Autodesk Inventor part; units mm, degrees
(part 2 of 2)
  line L934 (17.3523, 0.525) -> (17.2918, 0.4645)
  line L935 (17.2918, 0.4645) -> (17.2697, 0.3818)
  line L936 (17.2697, 0.3818) -> (17.2918, 0.2991)
  line L937 (17.2918, 0.2991) -> (17.3523, 0.2386)
  line L938 (17.3523, 0.2386) -> (17.435, 0.2164)
  line L939 (17.435, 0.2164) -> (17.5177, 0.2386)
  line L940 (17.5177, 0.2386) -> (17.5782, 0.2991)
  line L941 (17.5782, 0.2991) -> (17.6003, 0.3818)
  line L942 (14.4188, -4.4542) -> (14.3966, -4.3715)
  line L943 (14.3966, -4.3715) -> (14.3361, -4.311)
  line L944 (14.3361, -4.311) -> (14.2534, -4.2889)
  line L945 (14.2534, -4.2889) -> (14.1708, -4.311)
  line L946 (14.1708, -4.311) -> (14.1102, -4.3715)
  line L947 (14.1102, -4.3715) -> (14.0881, -4.4542)
  line L948 (14.0881, -4.4542) -> (14.1102, -4.5369)
  line L949 (14.1102, -4.5369) -> (14.1708, -4.5974)
  line L950 (14.1708, -4.5974) -> (14.2534, -4.6195)
  line L951 (14.2534, -4.6195) -> (14.3361, -4.5974)
  line L952 (14.3361, -4.5974) -> (14.3966, -4.5369)
  line L953 (14.3966, -4.5369) -> (14.4188, -4.4542)
  line L954 (17.4731, -10.5628) -> (17.4509, -10.4801)
  line L955 (17.4509, -10.4801) -> (17.3904, -10.4196)
  line L956 (17.3904, -10.4196) -> (17.3077, -10.3975)
  line L957 (17.3077, -10.3975) -> (17.2251, -10.4196)
  line L958 (17.2251, -10.4196) -> (17.1645, -10.4801)
  line L959 (17.1645, -10.4801) -> (17.1424, -10.5628)
  line L960 (17.1424, -10.5628) -> (17.1645, -10.6455)
  line L961 (17.1645, -10.6455) -> (17.2251, -10.706)
  line L962 (17.2251, -10.706) -> (17.3077, -10.7282)
  line L963 (17.3077, -10.7282) -> (17.3904, -10.706)
  line L964 (17.3904, -10.706) -> (17.4509, -10.6455)
  line L965 (17.4509, -10.6455) -> (17.4731, -10.5628)
  line L966 (14.546, -12.599) -> (14.5239, -12.5163)
  line L967 (14.5239, -12.5163) -> (14.4634, -12.4558)
  line L968 (14.4634, -12.4558) -> (14.3807, -12.4337)
  line L969 (14.3807, -12.4337) -> (14.298, -12.4558)
  line L970 (14.298, -12.4558) -> (14.2375, -12.5163)
  line L971 (14.2375, -12.5163) -> (14.2154, -12.599)
  line L972 (14.2154, -12.599) -> (14.2375, -12.6817)
  line L973 (14.2375, -12.6817) -> (14.298, -12.7422)
  line L974 (14.298, -12.7422) -> (14.3807, -12.7644)
  line L975 (14.3807, -12.7644) -> (14.4634, -12.7422)
  line L976 (14.4634, -12.7422) -> (14.5239, -12.6817)
  line L977 (14.5239, -12.6817) -> (14.546, -12.599)
  line L978 (15.5706, -6.8563) -> (15.5101, -6.9168)
  line L979 (15.5101, -6.9168) -> (15.488, -6.9995)
  line L980 (15.488, -6.9995) -> (15.5101, -7.0821)
  line L981 (15.5101, -7.0821) -> (15.5706, -7.1426)
  line L982 (15.5706, -7.1426) -> (15.6533, -7.1648)
  line L983 (15.6533, -7.1648) -> (15.736, -7.1426)
  line L984 (15.736, -7.1426) -> (15.7965, -7.0821)
  line L985 (15.7965, -7.0821) -> (15.8187, -6.9995)
  line L986 (17.0913, -12.09) -> (17.0691, -12.0073)
  line L987 (17.0691, -12.0073) -> (17.0086, -11.9468)
  line L988 (17.0086, -11.9468) -> (16.9259, -11.9246)
  line L989 (16.9259, -11.9246) -> (16.8433, -11.9468)
  line L990 (16.8433, -11.9468) -> (16.7828, -12.0073)
  line L991 (16.7828, -12.0073) -> (16.7606, -12.09)
  line L992 (16.7606, -12.09) -> (16.7828, -12.1726)
  line L993 (16.7828, -12.1726) -> (16.8433, -12.2332)
  line L994 (16.8433, -12.2332) -> (16.9259, -12.2553)
  line L995 (16.9259, -12.2553) -> (17.0086, -12.2332)
  line L996 (17.0086, -12.2332) -> (17.0691, -12.1726)
  line L997 (17.0691, -12.1726) -> (17.0913, -12.09)
  line L998 (17.3458, -13.6171) -> (17.3237, -13.5344)
  line L999 (17.3237, -13.5344) -> (17.2631, -13.4739)
  line L1000 (17.2631, -13.4739) -> (17.1805, -13.4518)
  line L1001 (17.1805, -13.4518) -> (17.0978, -13.4739)
  line L1002 (17.0978, -13.4739) -> (17.0373, -13.5344)
  line L1003 (17.0373, -13.5344) -> (17.0151, -13.6171)
  line L1004 (17.0151, -13.6171) -> (17.0373, -13.6998)
  line L1005 (17.0373, -13.6998) -> (17.0978, -13.7603)
  line L1006 (17.0978, -13.7603) -> (17.1805, -13.7825)
  line L1007 (17.1805, -13.7825) -> (17.2631, -13.7603)
  line L1008 (17.2631, -13.7603) -> (17.3237, -13.6998)
  line L1009 (17.3237, -13.6998) -> (17.3458, -13.6171)
  line L1010 (11.2372, -15.3988) -> (11.215, -15.3161)
  line L1011 (11.215, -15.3161) -> (11.1545, -15.2556)
  line L1012 (11.1545, -15.2556) -> (11.0719, -15.2335)
  line L1013 (11.0719, -15.2335) -> (10.9892, -15.2556)
  line L1014 (10.9892, -15.2556) -> (10.9287, -15.3161)
  line L1015 (10.9287, -15.3161) -> (10.9065, -15.3988)
  line L1016 (10.9065, -15.3988) -> (10.9287, -15.4815)
  line L1017 (10.9287, -15.4815) -> (10.9892, -15.542)
  line L1018 (10.9892, -15.542) -> (11.0719, -15.5641)
  line L1019 (11.0719, -15.5641) -> (11.1545, -15.542)
  line L1020 (11.1545, -15.542) -> (11.215, -15.4815)
  line L1021 (11.215, -15.4815) -> (11.2372, -15.3988)
  line L1022 (6.6557, -17.435) -> (6.6336, -17.3523)
  line L1023 (6.6336, -17.3523) -> (6.5731, -17.2918)
  line L1024 (6.5731, -17.2918) -> (6.4904, -17.2697)
  line L1025 (6.4904, -17.2697) -> (6.4077, -17.2918)
  line L1026 (6.4077, -17.2918) -> (6.3472, -17.3523)
  line L1027 (6.3472, -17.3523) -> (6.3251, -17.435)
  line L1028 (6.3251, -17.435) -> (6.3472, -17.5177)
  line L1029 (6.3472, -17.5177) -> (6.4077, -17.5782)
  line L1030 (6.4077, -17.5782) -> (6.4904, -17.6003)
  line L1031 (6.4904, -17.6003) -> (6.5731, -17.5782)
  line L1032 (6.5731, -17.5782) -> (6.6336, -17.5177)
  line L1033 (6.6336, -17.5177) -> (6.6557, -17.435)
  line L1034 (4.1105, -17.435) -> (4.0883, -17.3523)
  line L1035 (4.0883, -17.3523) -> (4.0278, -17.2918)
  line L1036 (4.0278, -17.2918) -> (3.9451, -17.2697)
  line L1037 (3.9451, -17.2697) -> (3.8625, -17.2918)
  line L1038 (3.8625, -17.2918) -> (3.802, -17.3523)
  line L1039 (3.802, -17.3523) -> (3.7798, -17.435)
  line L1040 (3.7798, -17.435) -> (3.802, -17.5177)
  line L1041 (3.802, -17.5177) -> (3.8625, -17.5782)
  line L1042 (3.8625, -17.5782) -> (3.9451, -17.6003)
  line L1043 (3.9451, -17.6003) -> (4.0278, -17.5782)
  line L1044 (4.0278, -17.5782) -> (4.0883, -17.5177)
  line L1045 (4.0883, -17.5177) -> (4.1105, -17.435)
  line L1046 (1.7976, -17.3523) -> (1.7371, -17.2918)
  line L1047 (1.7371, -17.2918) -> (1.6544, -17.2697)
  line L1048 (1.6544, -17.2697) -> (1.5717, -17.2918)
  line L1049 (1.5717, -17.2918) -> (1.5112, -17.3523)
  line L1050 (1.5112, -17.3523) -> (1.4891, -17.435)
  line L1051 (1.4891, -17.435) -> (1.5112, -17.5177)
  line L1052 (1.5112, -17.5177) -> (1.5717, -17.5782)
  line L1053 (1.5717, -17.5782) -> (1.6544, -17.6003)
  line L1054 (1.6544, -17.6003) -> (1.7371, -17.5782)
  line L1055 (1.7371, -17.5782) -> (1.7976, -17.5177)
  line L1056 (1.7976, -17.5177) -> (1.8198, -17.435)
  line L1057 (-4.117, -17.5782) -> (-4.0565, -17.5177)
  line L1058 (-4.0565, -17.5177) -> (-4.0343, -17.435)
  line L1059 (-1.7436, -17.435) -> (-1.7658, -17.3523)
  line L1060 (-1.7658, -17.3523) -> (-1.8263, -17.2918)
  line L1061 (-1.8263, -17.2918) -> (-1.9089, -17.2697)
  line L1062 (-1.9089, -17.2697) -> (-1.9916, -17.2918)
  line L1063 (-1.9916, -17.2918) -> (-2.0521, -17.3523)
  line L1064 (-2.0521, -17.3523) -> (-2.0743, -17.435)
  line L1065 (-2.0743, -17.435) -> (-2.0521, -17.5177)
  line L1066 (-2.0521, -17.5177) -> (-1.9916, -17.5782)
  line L1067 (-1.9916, -17.5782) -> (-1.9089, -17.6003)
  line L1068 (-1.9089, -17.6003) -> (-1.8263, -17.5782)
  line L1069 (-1.8263, -17.5782) -> (-1.7658, -17.5177)
  line L1070 (-1.7658, -17.5177) -> (-1.7436, -17.435)
  line L1071 (-5.816, -15.6533) -> (-5.8382, -15.5706)
  line L1072 (-5.8382, -15.5706) -> (-5.8987, -15.5101)
  line L1073 (-5.8987, -15.5101) -> (-5.9813, -15.488)
  line L1074 (-5.9813, -15.488) -> (-6.064, -15.5101)
  line L1075 (-6.064, -15.5101) -> (-6.1245, -15.5706)
  line L1076 (-6.1245, -15.5706) -> (-6.1467, -15.6533)
  line L1077 (-6.1467, -15.6533) -> (-6.1245, -15.736)
  line L1078 (-6.1245, -15.736) -> (-6.064, -15.7965)
  line L1079 (-6.064, -15.7965) -> (-5.9813, -15.8187)
  line L1080 (-5.9813, -15.8187) -> (-5.8987, -15.7965)
  line L1081 (-5.8987, -15.7965) -> (-5.8382, -15.736)
  line L1082 (-5.8382, -15.736) -> (-5.816, -15.6533)
  line L1083 (-8.8703, -14.8897) -> (-8.8925, -14.8071)
  line L1084 (-8.8925, -14.8071) -> (-8.953, -14.7466)
  line L1085 (-8.953, -14.7466) -> (-9.0357, -14.7244)
  line L1086 (-9.0357, -14.7244) -> (-9.1183, -14.7466)
  line L1087 (-9.1183, -14.7466) -> (-9.1788, -14.8071)
  line L1088 (-9.201, -14.8897) -> (-9.1788, -14.9724)
  line L1089 (-9.1788, -14.9724) -> (-9.1183, -15.0329)
  line L1090 (-9.1183, -15.0329) -> (-9.0357, -15.0551)
  line L1091 (-9.0357, -15.0551) -> (-8.953, -15.0329)
  line L1092 (-8.953, -15.0329) -> (-8.8925, -14.9724)
  line L1093 (-8.8925, -14.9724) -> (-8.8703, -14.8897)
  line L1094 (-11.6701, -14.8897) -> (-11.6922, -14.8071)
  line L1095 (-11.6922, -14.8071) -> (-11.7528, -14.7466)
  line L1096 (-11.7528, -14.7466) -> (-11.8354, -14.7244)
  line L1097 (-11.8354, -14.7244) -> (-11.9181, -14.7466)
  line L1098 (-11.9181, -14.7466) -> (-11.9786, -14.8071)
  line L1099 (-11.9786, -14.8071) -> (-12.0008, -14.8897)
  line L1100 (-12.0008, -14.8897) -> (-11.9786, -14.9724)
  line L1101 (-11.9786, -14.9724) -> (-11.9181, -15.0329)
  line L1102 (-11.9181, -15.0329) -> (-11.8354, -15.0551)
  line L1103 (-11.8354, -15.0551) -> (-11.7528, -15.0329)
  line L1104 (-11.7528, -15.0329) -> (-11.6922, -14.9724)
  line L1105 (-11.6922, -14.9724) -> (-11.6701, -14.8897)
  line L1106 (-13.4739, -15.8252) -> (-13.5344, -15.7647)
  line L1107 (-13.6998, -15.7647) -> (-13.7603, -15.8252)
  line L1108 (-13.7603, -15.8252) -> (-13.7825, -15.9078)
  line L1109 (-13.7825, -15.9078) -> (-13.7603, -15.9905)
  line L1110 (-13.7603, -15.9905) -> (-13.6998, -16.051)
  line L1111 (-13.6998, -16.051) -> (-13.6171, -16.0732)
  line L1112 (-13.6171, -16.0732) -> (-13.5344, -16.051)
  line L1113 (-13.5344, -16.051) -> (-13.4739, -15.9905)
  line L1114 (-13.4739, -15.9905) -> (-13.4518, -15.9078)
  line L1115 (-14.9789, -17.3077) -> (-15.0011, -17.2251)
  line L1116 (-15.0011, -17.2251) -> (-15.0616, -17.1645)
  line L1117 (-15.0616, -17.1645) -> (-15.1443, -17.1424)
  line L1118 (-15.1443, -17.1424) -> (-15.2269, -17.1645)
  line L1119 (-15.2269, -17.1645) -> (-15.2875, -17.2251)
  line L1120 (-15.2875, -17.2251) -> (-15.3096, -17.3077)
  line L1121 (-15.3096, -17.3077) -> (-15.2875, -17.3904)
  line L1122 (-15.2875, -17.3904) -> (-15.2269, -17.4509)
  line L1123 (-15.2269, -17.4509) -> (-15.1443, -17.4731)
  line L1124 (-15.1443, -17.4731) -> (-15.0616, -17.4509)
  line L1125 (-15.0616, -17.4509) -> (-15.0011, -17.3904)
  line L1126 (-15.0011, -17.3904) -> (-14.9789, -17.3077)
  line L1127 (-17.5177, -14.6193) -> (-17.5782, -14.6798)
  line L1128 (-17.5782, -14.6798) -> (-17.6003, -14.7625)
  line L1129 (-17.5782, -14.8452) -> (-17.5177, -14.9057)
  line L1130 (-17.5177, -14.9057) -> (-17.435, -14.9278)
  line L1131 (-17.435, -14.9278) -> (-17.3523, -14.9057)
  line L1132 (-17.3523, -14.9057) -> (-17.2918, -14.8452)
  line L1133 (-17.2918, -14.8452) -> (-17.2697, -14.7625)
  line L1134 (-15.488, -13.3626) -> (-15.5101, -13.2799)
  line L1135 (-15.5101, -13.2799) -> (-15.5706, -13.2194)
  line L1136 (-15.5706, -13.2194) -> (-15.6533, -13.1972)
  line L1137 (-15.6533, -13.1972) -> (-15.736, -13.2194)
  line L1138 (-15.736, -13.2194) -> (-15.7965, -13.2799)
  line L1139 (-15.7965, -13.2799) -> (-15.8187, -13.3626)
  line L1140 (-15.8187, -13.3626) -> (-15.7965, -13.4453)
  line L1141 (-15.6533, -13.5279) -> (-15.5706, -13.5058)
  line L1142 (-15.5706, -13.5058) -> (-15.5101, -13.4453)
  line L1143 (-15.5101, -13.4453) -> (-15.488, -13.3626)
  line L1144 (-14.9789, -11.5809) -> (-15.0011, -11.4982)
  line L1145 (-15.0011, -11.4982) -> (-15.0616, -11.4377)
  line L1146 (-15.0616, -11.4377) -> (-15.1443, -11.4156)
  line L1147 (-15.1443, -11.4156) -> (-15.2269, -11.4377)
  line L1148 (-15.2269, -11.4377) -> (-15.2875, -11.4982)
  line L1149 (-15.2875, -11.4982) -> (-15.3096, -11.5809)
  line L1150 (-15.3096, -11.5809) -> (-15.2875, -11.6636)
  line L1151 (-15.2875, -11.6636) -> (-15.2269, -11.7241)
  line L1152 (-15.2269, -11.7241) -> (-15.1443, -11.7463)
  line L1153 (-15.1443, -11.7463) -> (-15.0616, -11.7241)
  line L1154 (-15.0616, -11.7241) -> (-15.0011, -11.6636)
  line L1155 (-15.0011, -11.6636) -> (-14.9789, -11.5809)
  line L1156 (-14.7244, -8.7811) -> (-14.7466, -8.6985)
  line L1157 (-14.7466, -8.6985) -> (-14.8071, -8.6379)
  line L1158 (-14.8071, -8.6379) -> (-14.8897, -8.6158)
  line L1159 (-14.8897, -8.6158) -> (-14.9724, -8.6379)
  line L1160 (-14.9724, -8.6379) -> (-15.0329, -8.6985)
  line L1161 (-15.0329, -8.6985) -> (-15.0551, -8.7811)
  line L1162 (-15.0551, -8.7811) -> (-15.0329, -8.8638)
  line L1163 (-15.0329, -8.8638) -> (-14.9724, -8.9243)
  line L1164 (-14.9724, -8.9243) -> (-14.8897, -8.9465)
  line L1165 (-14.8897, -8.9465) -> (-14.8071, -8.9243)
  line L1166 (-14.8071, -8.9243) -> (-14.7466, -8.8638)
  line L1167 (-14.7466, -8.8638) -> (-14.7244, -8.7811)
  line L1168 (-15.488, -6.2359) -> (-15.5101, -6.1532)
  line L1169 (-15.5101, -6.1532) -> (-15.5706, -6.0927)
  line L1170 (-15.5706, -6.0927) -> (-15.6533, -6.0705)
  line L1171 (-15.6533, -6.0705) -> (-15.736, -6.0927)
  line L1172 (-15.736, -6.0927) -> (-15.7965, -6.1532)
  line L1173 (-15.7965, -6.1532) -> (-15.8187, -6.2359)
  line L1174 (-15.8187, -6.2359) -> (-15.7965, -6.3185)
  line L1175 (-15.7965, -6.3185) -> (-15.736, -6.3791)
  line L1176 (-15.736, -6.3791) -> (-15.6533, -6.4012)
  line L1177 (-15.6533, -6.4012) -> (-15.5706, -6.3791)
  line L1178 (-15.5706, -6.3791) -> (-15.5101, -6.3185)
  line L1179 (-15.5101, -6.3185) -> (-15.488, -6.2359)
  line L1180 (-17.2697, -1.6544) -> (-17.2918, -1.5717)
  line L1181 (-17.2918, -1.5717) -> (-17.3523, -1.5112)
  line L1182 (-17.3523, -1.5112) -> (-17.435, -1.4891)
  line L1183 (-17.435, -1.4891) -> (-17.5177, -1.5112)
  line L1184 (-17.5177, -1.5112) -> (-17.5782, -1.5717)
  line L1185 (-17.5782, -1.5717) -> (-17.6003, -1.6544)
  line L1186 (-17.6003, -1.6544) -> (-17.5782, -1.7371)
  line L1187 (-17.5782, -1.7371) -> (-17.5177, -1.7976)
  line L1188 (-17.5177, -1.7976) -> (-17.435, -1.8198)
  line L1189 (-17.435, -1.8198) -> (-17.3523, -1.7976)
  line L1190 (-17.3523, -1.7976) -> (-17.2918, -1.7371)
  line L1191 (-17.2918, -1.7371) -> (-17.2697, -1.6544)
  line L1192 (-17.2697, 0.8908) -> (-17.2918, 0.9735)
  line L1193 (-17.2918, 0.9735) -> (-17.3523, 1.034)
  line L1194 (-17.3523, 1.034) -> (-17.435, 1.0562)
  line L1195 (-17.435, 1.0562) -> (-17.5177, 1.034)
  line L1196 (-17.5177, 1.034) -> (-17.5782, 0.9735)
  line L1197 (-17.5782, 0.9735) -> (-17.6003, 0.8908)
  line L1198 (-17.6003, 0.8908) -> (-17.5782, 0.8082)
  line L1199 (-17.5782, 0.8082) -> (-17.5177, 0.7476)
  line L1200 (-17.5177, 0.7476) -> (-17.435, 0.7255)
  line L1201 (-17.435, 0.7255) -> (-17.3523, 0.7476)
  line L1202 (-17.3523, 0.7476) -> (-17.2918, 0.8082)
  line L1203 (-17.2918, 0.8082) -> (-17.2697, 0.8908)
  line L1204 (-17.2697, 3.6906) -> (-17.2918, 3.7733)
  line L1205 (-17.2918, 3.7733) -> (-17.3523, 3.8338)
  line L1206 (-17.3523, 3.8338) -> (-17.435, 3.856)
  line L1207 (-17.435, 3.856) -> (-17.5177, 3.8338)
  line L1208 (-17.5177, 3.8338) -> (-17.5782, 3.7733)
  line L1209 (-17.5782, 3.7733) -> (-17.6003, 3.6906)
  line L1210 (-17.6003, 3.6906) -> (-17.5782, 3.6079)
  line L1211 (-17.5782, 3.6079) -> (-17.5177, 3.5474)
  line L1212 (-17.5177, 3.5474) -> (-17.435, 3.5253)
  line L1213 (-17.435, 3.5253) -> (-17.3523, 3.5474)
  line L1214 (-17.3523, 3.5474) -> (-17.2918, 3.6079)
  line L1215 (-17.2918, 3.6079) -> (-17.2697, 3.6906)
  line L1216 (-17.2697, 6.7449) -> (-17.2918, 6.8276)
  line L1217 (-17.3523, 6.8881) -> (-17.435, 6.9103)
  line L1218 (-17.5177, 6.8881) -> (-17.5782, 6.8276)
  line L1219 (-17.5782, 6.8276) -> (-17.6003, 6.7449)
  line L1220 (-17.6003, 6.7449) -> (-17.5782, 6.6623)
  line L1221 (-17.5782, 6.6623) -> (-17.5177, 6.6017)
  line L1222 (-17.5177, 6.6017) -> (-17.435, 6.5796)
  line L1223 (-17.435, 6.5796) -> (-17.3523, 6.6017)
  line L1224 (-17.3523, 6.6017) -> (-17.2918, 6.6623)
  line L1225 (-17.2918, 6.6623) -> (-17.2697, 6.7449)
  line L1226 (-17.2697, 9.2902) -> (-17.2918, 9.3729)
  line L1227 (-17.2918, 9.3729) -> (-17.3523, 9.4334)
  line L1228 (-17.3523, 9.4334) -> (-17.435, 9.4555)
  line L1229 (-17.435, 9.4555) -> (-17.5177, 9.4334)
  line L1230 (-17.5177, 9.4334) -> (-17.5782, 9.3729)
  line L1231 (-17.5782, 9.3729) -> (-17.6003, 9.2902)
  line L1232 (-17.6003, 9.2902) -> (-17.5782, 9.2075)
  line L1233 (-17.5782, 9.2075) -> (-17.5177, 9.147)
  line L1234 (-17.5177, 9.147) -> (-17.435, 9.1248)
  line L1235 (-17.435, 9.1248) -> (-17.3523, 9.147)
  line L1236 (-17.3523, 9.147) -> (-17.2918, 9.2075)
  line L1237 (-17.2918, 9.2075) -> (-17.2697, 9.2902)
  line L1238 (-17.2697, 11.5809) -> (-17.2918, 11.6636)
  line L1239 (-17.2918, 11.6636) -> (-17.3523, 11.7241)
  line L1240 (-17.3523, 11.7241) -> (-17.435, 11.7463)
  line L1241 (-17.5177, 11.7241) -> (-17.5782, 11.6636)
  line L1242 (-17.5782, 11.6636) -> (-17.6003, 11.5809)
  line L1243 (-17.6003, 11.5809) -> (-17.5782, 11.4982)
  line L1244 (-17.5782, 11.4982) -> (-17.5177, 11.4377)
  line L1245 (-17.5177, 11.4377) -> (-17.435, 11.4156)
  line L1246 (-17.435, 11.4156) -> (-17.3523, 11.4377)
  line L1247 (-17.3523, 11.4377) -> (-17.2918, 11.4982)
  line L1248 (-17.2918, 11.4982) -> (-17.2697, 11.5809)
  line L1249 (-17.0151, 12.8535) -> (-17.0373, 12.9362)
  line L1250 (-17.0373, 12.9362) -> (-17.0978, 12.9967)
  line L1251 (-17.0978, 12.9967) -> (-17.1805, 13.0189)
  line L1252 (-17.1805, 13.0189) -> (-17.2631, 12.9967)
  line L1253 (-17.2631, 12.9967) -> (-17.3237, 12.9362)
  line L1254 (-17.3237, 12.9362) -> (-17.3458, 12.8535)
  line L1255 (-17.3458, 12.8535) -> (-17.3237, 12.7709)
  line L1256 (-17.3237, 12.7709) -> (-17.2631, 12.7103)
  line L1257 (-17.2631, 12.7103) -> (-17.1805, 12.6882)
  line L1258 (-17.1805, 12.6882) -> (-17.0978, 12.7103)
  line L1259 (-17.0978, 12.7103) -> (-17.0373, 12.7709)
  line L1260 (-17.0373, 12.7709) -> (-17.0151, 12.8535)
  line L1261 (-15.7425, 13.1081) -> (-15.7647, 13.1907)
  line L1262 (-15.7647, 13.1907) -> (-15.8252, 13.2513)
  line L1263 (-15.8252, 13.2513) -> (-15.9078, 13.2734)
  line L1264 (-15.9078, 13.2734) -> (-15.9905, 13.2513)
  line L1265 (-15.9905, 13.2513) -> (-16.051, 13.1907)
  line L1266 (-16.051, 13.1907) -> (-16.0732, 13.1081)
  line L1267 (-16.0732, 13.1081) -> (-16.051, 13.0254)
  line L1268 (-16.051, 13.0254) -> (-15.9905, 12.9649)
  line L1269 (-15.9905, 12.9649) -> (-15.9078, 12.9427)
  line L1270 (-15.8252, 12.9649) -> (-15.7647, 13.0254)
  line L1271 (-15.7647, 13.0254) -> (-15.7425, 13.1081)
  line L1272 (-12.7709, 17.5782) -> (-12.8535, 17.6003)
  line L1273 (-12.8535, 17.6003) -> (-12.9362, 17.5782)
  line L1274 (-12.9362, 17.5782) -> (-12.9967, 17.5177)
  line L1275 (-12.9967, 17.5177) -> (-13.0189, 17.435)
  line L1276 (-13.0189, 17.435) -> (-12.9967, 17.3523)
  line L1277 (-12.9967, 17.3523) -> (-12.9362, 17.2918)
  line L1278 (-12.8535, 17.2697) -> (-12.7709, 17.2918)
  line L1279 (-16.2516, 5.4723) -> (-16.2737, 5.555)
  line L1280 (-16.2737, 5.555) -> (-16.3342, 5.6155)
  line L1281 (-16.3342, 5.6155) -> (-16.4169, 5.6376)
  line L1282 (-16.4169, 5.6376) -> (-16.4996, 5.6155)
  line L1283 (-16.4996, 5.6155) -> (-16.5601, 5.555)
  line L1284 (-16.5601, 5.555) -> (-16.5822, 5.4723)
  line L1285 (-16.5822, 5.4723) -> (-16.5601, 5.3896)
  line L1286 (-16.4996, 5.3291) -> (-16.4169, 5.307)
  line L1287 (-16.3342, 5.3291) -> (-16.2737, 5.3896)
  line L1288 (-16.2737, 5.3896) -> (-16.2516, 5.4723)
  line L1289 (-15.997, 11.8354) -> (-16.0192, 11.9181)
  line L1290 (-16.0192, 11.9181) -> (-16.0797, 11.9786)
  line L1291 (-16.0797, 11.9786) -> (-16.1624, 12.0008)
  line L1292 (-16.1624, 12.0008) -> (-16.245, 11.9786)
  line L1293 (-16.245, 11.9786) -> (-16.3056, 11.9181)
  line L1294 (-16.3056, 11.9181) -> (-16.3277, 11.8354)
  line L1295 (-16.3277, 11.8354) -> (-16.3056, 11.7528)
  line L1296 (-16.3056, 11.7528) -> (-16.245, 11.6922)
  line L1297 (-16.245, 11.6922) -> (-16.1624, 11.6701)
  line L1298 (-16.1624, 11.6701) -> (-16.0797, 11.6922)
  line L1299 (-16.0797, 11.6922) -> (-16.0192, 11.7528)
  line L1300 (-16.0192, 11.7528) -> (-15.997, 11.8354)
  line L1301 (-6.6336, 14.1708) -> (-6.5731, 14.1102)
  line L1302 (-6.4077, 14.1102) -> (-6.3472, 14.1708)
  line L1303 (-5.307, 13.9989) -> (-5.3291, 14.0816)
  line L1304 (-5.4723, 14.1642) -> (-5.555, 14.1421)
  line L1305 (-5.6376, 13.9989) -> (-5.6155, 13.9162)
  line L1306 (-5.555, 13.8557) -> (-5.4723, 13.8336)
  line L1307 (-5.4723, 13.8336) -> (-5.3896, 13.8557)
  line L1308 (-0.7476, 17.5177) -> (-0.8082, 17.5782)
  line L1309 (-0.8082, 17.5782) -> (-0.8908, 17.6003)
  line L1310 (-0.8908, 17.6003) -> (-0.9735, 17.5782)
  line L1311 (-0.9735, 17.5782) -> (-1.034, 17.5177)
  line L1312 (-1.034, 17.5177) -> (-1.0562, 17.435)
  line L1313 (-1.0562, 17.435) -> (-1.034, 17.3523)
  line L1314 (-1.034, 17.3523) -> (-0.9735, 17.2918)
  line L1315 (-0.9735, 17.2918) -> (-0.8908, 17.2697)
  line L1316 (-0.8908, 17.2697) -> (-0.8082, 17.2918)
  line L1317 (-0.8082, 17.2918) -> (-0.7476, 17.3523)
  line L1318 (-0.7476, 17.3523) -> (-0.7255, 17.435)
  line L1319 (1.0562, 17.435) -> (1.034, 17.5177)
  line L1320 (1.034, 17.5177) -> (0.9735, 17.5782)
  line L1321 (0.9735, 17.5782) -> (0.8908, 17.6003)
  line L1322 (0.8908, 17.6003) -> (0.8082, 17.5782)
  line L1323 (0.8082, 17.5782) -> (0.7476, 17.5177)
  line L1324 (0.7476, 17.5177) -> (0.7255, 17.435)
  line L1325 (0.7255, 17.435) -> (0.7476, 17.3523)
  line L1326 (0.7476, 17.3523) -> (0.8082, 17.2918)
  line L1327 (0.8082, 17.2918) -> (0.8908, 17.2697)
  line L1328 (0.8908, 17.2697) -> (0.9735, 17.2918)
  line L1329 (0.9735, 17.2918) -> (1.034, 17.3523)
  line L1330 (1.034, 17.3523) -> (1.0562, 17.435)
  line L1331 (7.6738, 16.6714) -> (7.6517, 16.7541)
  line L1332 (7.6517, 16.7541) -> (7.5912, 16.8146)
  line L1333 (7.5912, 16.8146) -> (7.5085, 16.8368)
  line L1334 (7.5085, 16.8368) -> (7.4258, 16.8146)
  line L1335 (7.4258, 16.8146) -> (7.3653, 16.7541)
  line L1336 (7.3653, 16.7541) -> (7.3432, 16.6714)
  line L1337 (7.3432, 16.6714) -> (7.3653, 16.5888)
  line L1338 (7.3653, 16.5888) -> (7.4258, 16.5282)
  line L1339 (7.4258, 16.5282) -> (7.5085, 16.5061)
  line L1340 (7.5085, 16.5061) -> (7.5912, 16.5282)
  line L1341 (7.5912, 16.5282) -> (7.6517, 16.5888)
  line L1342 (7.6517, 16.5888) -> (7.6738, 16.6714)
  line L1343 (3.6014, 16.4169) -> (3.5793, 16.4996)
  line L1344 (3.5793, 16.4996) -> (3.5188, 16.5601)
  line L1345 (3.5188, 16.5601) -> (3.4361, 16.5822)
  line L1346 (3.4361, 16.5822) -> (3.3534, 16.5601)
  line L1347 (3.3534, 16.5601) -> (3.2929, 16.4996)
  line L1348 (3.2929, 16.4996) -> (3.2708, 16.4169)
  line L1349 (3.2708, 16.4169) -> (3.2929, 16.3342)
  line L1350 (3.2929, 16.3342) -> (3.3534, 16.2737)
  line L1351 (3.3534, 16.2737) -> (3.4361, 16.2516)
  line L1352 (3.4361, 16.2516) -> (3.5188, 16.2737)
  line L1353 (3.5188, 16.2737) -> (3.5793, 16.3342)
  line L1354 (3.5793, 16.3342) -> (3.6014, 16.4169)
  line L1355 (4.6195, 17.435) -> (4.5974, 17.5177)
  line L1356 (4.5974, 17.5177) -> (4.5369, 17.5782)
  line L1357 (4.5369, 17.5782) -> (4.4542, 17.6003)
  line L1358 (4.4542, 17.6003) -> (4.3715, 17.5782)
  line L1359 (4.3715, 17.5782) -> (4.311, 17.5177)
  line L1360 (4.311, 17.5177) -> (4.2889, 17.435)
  line L1361 (4.2889, 17.435) -> (4.311, 17.3523)
  line L1362 (4.311, 17.3523) -> (4.3715, 17.2918)
  line L1363 (4.3715, 17.2918) -> (4.4542, 17.2697)
  line L1364 (4.4542, 17.2697) -> (4.5369, 17.2918)
  line L1365 (4.5369, 17.2918) -> (4.5974, 17.3523)
  line L1366 (4.5974, 17.3523) -> (4.6195, 17.435)
  line L1367 (4.2823, 15.0011) -> (4.3429, 15.0616)
  line L1368 (15.5641, 10.5628) -> (15.542, 10.6455)
  line L1369 (15.542, 10.6455) -> (15.4815, 10.706)
  line L1370 (15.4815, 10.706) -> (15.3988, 10.7282)
  line L1371 (15.3988, 10.7282) -> (15.3161, 10.706)
  line L1372 (15.3161, 10.706) -> (15.2556, 10.6455)
  line L1373 (15.2556, 10.6455) -> (15.2335, 10.5628)
  line L1374 (15.2335, 10.5628) -> (15.2556, 10.4801)
  line L1375 (15.2556, 10.4801) -> (15.3161, 10.4196)
  line L1376 (15.3161, 10.4196) -> (15.3988, 10.3975)
  line L1377 (15.3988, 10.3975) -> (15.4815, 10.4196)
  line L1378 (15.4815, 10.4196) -> (15.542, 10.4801)
  line L1379 (15.542, 10.4801) -> (15.5641, 10.5628)
  line L1380 (14.546, 9.5447) -> (14.5239, 9.6274)
  line L1381 (14.5239, 9.6274) -> (14.4634, 9.6879)
  line L1382 (14.4634, 9.6879) -> (14.3807, 9.71)
  line L1383 (14.3807, 9.71) -> (14.298, 9.6879)
  line L1384 (14.298, 9.6879) -> (14.2375, 9.6274)
  line L1385 (14.2375, 9.6274) -> (14.2154, 9.5447)
  line L1386 (14.2154, 9.5447) -> (14.2375, 9.462)
  line L1387 (14.2375, 9.462) -> (14.298, 9.4015)
  line L1388 (14.298, 9.4015) -> (14.3807, 9.3794)
  line L1389 (14.3807, 9.3794) -> (14.4634, 9.4015)
  line L1390 (14.4634, 9.4015) -> (14.5239, 9.462)
  line L1391 (14.5239, 9.462) -> (14.546, 9.5447)
  line L1392 (2.3288, 16.9259) -> (2.3067, 17.0086)
  line L1393 (2.3067, 17.0086) -> (2.2461, 17.0691)
  line L1394 (2.2461, 17.0691) -> (2.1635, 17.0913)
  line L1395 (2.1635, 17.0913) -> (2.0808, 17.0691)
  line L1396 (2.0808, 17.0691) -> (2.0203, 17.0086)
  line L1397 (2.0203, 17.0086) -> (1.9981, 16.9259)
  line L1398 (1.9981, 16.9259) -> (2.0203, 16.8433)
  line L1399 (2.0203, 16.8433) -> (2.0808, 16.7828)
  line L1400 (2.0808, 16.7828) -> (2.1635, 16.7606)
  line L1401 (2.1635, 16.7606) -> (2.2461, 16.7828)
  line L1402 (2.2461, 16.7828) -> (2.3067, 16.8433)
  line L1403 (2.3067, 16.8433) -> (2.3288, 16.9259)
  line L1404 (13.6552, 10.4355) -> (13.633, 10.5182)
  line L1405 (13.633, 10.5182) -> (13.5725, 10.5787)
  line L1406 (13.5725, 10.5787) -> (13.4899, 10.6009)
  line L1407 (13.4899, 10.6009) -> (13.4072, 10.5787)
  line L1408 (13.4072, 10.5787) -> (13.3467, 10.5182)
  line L1409 (13.3467, 10.5182) -> (13.3245, 10.4355)
  line L1410 (13.3245, 10.4355) -> (13.3467, 10.3529)
  line L1411 (13.3467, 10.3529) -> (13.4072, 10.2924)
  line L1412 (13.4072, 10.2924) -> (13.4899, 10.2702)
  line L1413 (13.4899, 10.2702) -> (13.5725, 10.2924)
  line L1414 (13.5725, 10.2924) -> (13.633, 10.3529)
  line L1415 (13.633, 10.3529) -> (13.6552, 10.4355)
  line L1416 (14.2915, 3.6906) -> (14.2694, 3.7733)
  line L1417 (14.2694, 3.7733) -> (14.2088, 3.8338)
  line L1418 (14.2088, 3.8338) -> (14.1262, 3.856)
  line L1419 (14.1262, 3.856) -> (14.0435, 3.8338)
  line L1420 (14.0435, 3.8338) -> (13.983, 3.7733)
  line L1421 (13.983, 3.7733) -> (13.9608, 3.6906)
  line L1422 (13.9608, 3.6906) -> (13.983, 3.6079)
  line L1423 (13.983, 3.6079) -> (14.0435, 3.5474)
  line L1424 (14.0435, 3.5474) -> (14.1262, 3.5253)
  line L1425 (14.1262, 3.5253) -> (14.2088, 3.5474)
  line L1426 (14.2088, 3.5474) -> (14.2694, 3.6079)
  line L1427 (14.2694, 3.6079) -> (14.2915, 3.6906)
  line L1428 (12.7644, 3.0543) -> (12.7422, 3.137)
  line L1429 (12.7422, 3.137) -> (12.6817, 3.1975)
  line L1430 (12.6817, 3.1975) -> (12.599, 3.2196)
  line L1431 (12.599, 3.2196) -> (12.5163, 3.1975)
  line L1432 (12.5163, 3.1975) -> (12.4558, 3.137)
  line L1433 (12.4558, 3.137) -> (12.4337, 3.0543)
  line L1434 (12.4337, 3.0543) -> (12.4558, 2.9716)
  line L1435 (12.4558, 2.9716) -> (12.5163, 2.9111)
  line L1436 (12.5163, 2.9111) -> (12.599, 2.889)
  line L1437 (12.599, 2.889) -> (12.6817, 2.9111)
  line L1438 (12.6817, 2.9111) -> (12.7422, 2.9716)
  line L1439 (12.7422, 2.9716) -> (12.7644, 3.0543)
  line L1440 (-2.1794, 12.9362) -> (-2.2015, 12.8535)
  line L1441 (-2.2015, 12.8535) -> (-2.1794, 12.7709)
  line L1442 (-2.1794, 12.7709) -> (-2.1189, 12.7103)
  line L1443 (-2.1189, 12.7103) -> (-2.0362, 12.6882)
  line L1444 (-2.0362, 12.6882) -> (-1.9535, 12.7103)
  line L1445 (-1.9535, 12.7103) -> (-1.893, 12.7709)
  line L1446 (-1.893, 12.7709) -> (-1.8709, 12.8535)
  line L1447 (12.5098, -12.3445) -> (12.4877, -12.2618)
  line L1448 (12.4877, -12.2618) -> (12.4272, -12.2013)
  line L1449 (12.4272, -12.2013) -> (12.3445, -12.1791)
  line L1450 (12.2618, -12.2013) -> (12.2013, -12.2618)
  line L1451 (12.2013, -12.2618) -> (12.1791, -12.3445)
  line L1452 (12.1791, -12.3445) -> (12.2013, -12.4272)
  line L1453 (12.2013, -12.4272) -> (12.2618, -12.4877)
  line L1454 (12.2618, -12.4877) -> (12.3445, -12.5098)
  line L1455 (12.3445, -12.5098) -> (12.4272, -12.4877)
  line L1456 (12.4272, -12.4877) -> (12.4877, -12.4272)
  line L1457 (12.4877, -12.4272) -> (12.5098, -12.3445)
  line L1458 (4.6706, -14.3807) -> (4.6928, -14.4634)
  line L1459 (4.6928, -14.4634) -> (4.7533, -14.5239)
  line L1460 (4.7533, -14.5239) -> (4.836, -14.546)
  line L1461 (4.836, -14.546) -> (4.9187, -14.5239)
  line L1462 (4.9187, -14.5239) -> (4.9792, -14.4634)
  line L1463 (4.9792, -14.4634) -> (5.0013, -14.3807)
  line L1464 (-13.3245, -13.4899) -> (-13.3467, -13.4072)
  line L1465 (-13.3467, -13.4072) -> (-13.4072, -13.3467)
  line L1466 (-13.4072, -13.3467) -> (-13.4899, -13.3245)
  line L1467 (-13.4899, -13.3245) -> (-13.5725, -13.3467)
  line L1468 (-13.5725, -13.3467) -> (-13.633, -13.4072)
  line L1469 (-13.633, -13.4072) -> (-13.6552, -13.4899)
  line L1470 (-13.6552, -13.4899) -> (-13.633, -13.5725)
  line L1471 (-13.633, -13.5725) -> (-13.5725, -13.633)
  line L1472 (-13.5725, -13.633) -> (-13.4899, -13.6552)
  line L1473 (-13.4899, -13.6552) -> (-13.4072, -13.633)
  line L1474 (-13.4072, -13.633) -> (-13.3467, -13.5725)
  line L1475 (-13.3467, -13.5725) -> (-13.3245, -13.4899)
  line L1476 (-14.4634, 13.5058) -> (-14.5239, 13.4453)
  line L1477 (-14.5239, 13.4453) -> (-14.546, 13.3626)
  line L1478 (-14.546, 13.3626) -> (-14.5239, 13.2799)
  line L1479 (-14.5239, 13.2799) -> (-14.4634, 13.2194)
  line L1480 (-14.4634, 13.2194) -> (-14.3807, 13.1972)
  line L1481 (-14.3807, 13.1972) -> (-14.298, 13.2194)
  line L1482 (-14.298, 13.2194) -> (-14.2375, 13.2799)
  line L1483 (-14.2375, 13.2799) -> (-14.2154, 13.3626)
  line L1484 (-14.8517, 11.5809) -> (-14.8738, 11.6636)
  line L1485 (-14.8738, 11.6636) -> (-14.9343, 11.7241)
  line L1486 (-14.9343, 11.7241) -> (-15.017, 11.7463)
  line L1487 (-15.017, 11.7463) -> (-15.0997, 11.7241)
  line L1488 (-15.0997, 11.7241) -> (-15.1602, 11.6636)
  line L1489 (-15.1602, 11.6636) -> (-15.1823, 11.5809)
  line L1490 (-15.1823, 11.5809) -> (-15.1602, 11.4982)
  line L1491 (-15.1602, 11.4982) -> (-15.0997, 11.4377)
  line L1492 (-15.0997, 11.4377) -> (-15.017, 11.4156)
  line L1493 (-15.017, 11.4156) -> (-14.9343, 11.4377)
  line L1494 (-14.9343, 11.4377) -> (-14.8738, 11.4982)
  line L1495 (-14.8738, 11.4982) -> (-14.8517, 11.5809)
  line L1496 (-14.8517, 9.2902) -> (-14.8738, 9.3729)
  line L1497 (-14.8738, 9.3729) -> (-14.9343, 9.4334)
  line L1498 (-14.9343, 9.4334) -> (-15.017, 9.4555)
  line L1499 (-15.017, 9.4555) -> (-15.0997, 9.4334)
  line L1500 (-15.0997, 9.4334) -> (-15.1602, 9.3729)
  line L1501 (-15.1602, 9.3729) -> (-15.1823, 9.2902)
  line L1502 (-15.1823, 9.2902) -> (-15.1602, 9.2075)
  line L1503 (-15.1602, 9.2075) -> (-15.0997, 9.147)
  line L1504 (-15.0997, 9.147) -> (-15.017, 9.1248)
  line L1505 (-15.017, 9.1248) -> (-14.9343, 9.147)
  line L1506 (-14.8738, 9.2075) -> (-14.8517, 9.2902)
  line L1507 (17.6003, 4.5815) -> (17.5782, 4.6641)
  line L1508 (17.5782, 4.6641) -> (17.5177, 4.7246)
  line L1509 (17.5177, 4.7246) -> (17.435, 4.7468)
  line L1510 (17.435, 4.7468) -> (17.3523, 4.7246)
  line L1511 (17.3523, 4.7246) -> (17.2918, 4.6641)
  line L1512 (17.2918, 4.6641) -> (17.2697, 4.5815)
  line L1513 (17.2697, 4.5815) -> (17.2918, 4.4988)
  line L1514 (17.2918, 4.4988) -> (17.3523, 4.4383)
  line L1515 (17.3523, 4.4383) -> (17.435, 4.4161)
  line L1516 (17.435, 4.4161) -> (17.5177, 4.4383)
  line L1517 (17.5177, 4.4383) -> (17.5782, 4.4988)
  line L1518 (17.5782, 4.4988) -> (17.6003, 4.5815)
  line L1519 (1.6703, 3.646) -> (1.6098, 3.7065)
  line L1520 (1.6098, 3.7065) -> (1.5272, 3.7287)
  line L1521 (1.5272, 3.7287) -> (1.4445, 3.7065)
  line L1522 (1.4445, 3.7065) -> (1.384, 3.646)
  line L1523 (1.384, 3.646) -> (1.3618, 3.5634)
  line L1524 (1.3618, 3.5634) -> (1.384, 3.4807)
  line L1525 (1.384, 3.4807) -> (1.4445, 3.4202)
  line L1526 (1.4445, 3.4202) -> (1.5272, 3.398)
  line L1527 (1.5272, 3.398) -> (1.6098, 3.4202)
  line L1528 (1.6098, 3.4202) -> (1.6703, 3.4807)
  line L1529 (1.6703, 3.4807) -> (1.6925, 3.5634)
  line L1530 (5.2559, 0) -> (5.2337, 0.0827)
  line L1531 (5.2337, 0.0827) -> (5.1732, 0.1432)
  line L1532 (5.1732, 0.1432) -> (5.0905, 0.1653)
  line L1533 (5.0905, 0.1653) -> (5.0078, 0.1432)
  line L1534 (5.0078, 0.1432) -> (4.9473, 0.0827)
  line L1535 (4.9473, 0.0827) -> (4.9252, 0)
  line L1536 (4.9252, 0) -> (4.9473, -0.0827)
  line L1537 (4.9473, -0.0827) -> (5.0078, -0.1432)
  line L1538 (5.0078, -0.1432) -> (5.0905, -0.1653)
  line L1539 (5.0905, -0.1653) -> (5.1732, -0.1432)
  line L1540 (5.1732, -0.1432) -> (5.2337, -0.0827)
  line L1541 (5.2337, -0.0827) -> (5.2559, 0)
  line L1542 (16.0797, -9.3061) -> (16.1624, -9.3283)
  line L1543 (16.3056, -9.2456) -> (16.3277, -9.1629)
  line L1544 (3.4742, 12.7263) -> (3.452, 12.8089)
  line L1545 (3.452, 12.8089) -> (3.3915, 12.8695)
  line L1546 (3.3915, 12.8695) -> (3.3088, 12.8916)
  line L1547 (3.3088, 12.8916) -> (3.2262, 12.8695)
  line L1548 (3.2262, 12.8695) -> (3.1656, 12.8089)
  line L1549 (3.1656, 12.8089) -> (3.1435, 12.7263)
  line L1550 (3.1435, 12.7263) -> (3.1656, 12.6436)
  line L1551 (3.1656, 12.6436) -> (3.2262, 12.5831)
  line L1552 (3.2262, 12.5831) -> (3.3088, 12.5609)
  line L1553 (3.3088, 12.5609) -> (3.3915, 12.5831)
  line L1554 (3.3915, 12.5831) -> (3.452, 12.6436)
  line L1555 (3.452, 12.6436) -> (3.4742, 12.7263)
  line L1556 (2.5833, 11.8354) -> (2.5612, 11.9181)
  line L1557 (2.5007, 11.9786) -> (2.418, 12.0008)
  line L1558 (2.418, 12.0008) -> (2.3353, 11.9786)
  line L1559 (2.3353, 11.9786) -> (2.2748, 11.9181)
  line L1560 (2.2748, 11.9181) -> (2.2527, 11.8354)
  line L1561 (2.2527, 11.8354) -> (2.2748, 11.7528)
  line L1562 (2.2748, 11.7528) -> (2.3353, 11.6922)
  line L1563 (2.3353, 11.6922) -> (2.418, 11.6701)
  line L1564 (2.418, 11.6701) -> (2.5007, 11.6922)
  line L1565 (2.5007, 11.6922) -> (2.5612, 11.7528)
  line L1566 (2.5612, 11.7528) -> (2.5833, 11.8354)
  line L1567 (-4.1616, 12.9808) -> (-4.1837, 13.0635)
  line L1568 (-4.1837, 13.0635) -> (-4.2443, 13.124)
  line L1569 (-4.2443, 13.124) -> (-4.3269, 13.1461)
  line L1570 (-4.3269, 13.1461) -> (-4.4096, 13.124)
  line L1571 (-4.4096, 13.124) -> (-4.4701, 13.0635)
  line L1572 (-4.4701, 13.0635) -> (-4.4923, 12.9808)
  line L1573 (-4.4923, 12.9808) -> (-4.4701, 12.8981)
  line L1574 (-4.4701, 12.8981) -> (-4.4096, 12.8376)
  line L1575 (-4.4096, 12.8376) -> (-4.3269, 12.8155)
  line L1576 (-4.3269, 12.8155) -> (-4.2443, 12.8376)
  line L1577 (-4.2443, 12.8376) -> (-4.1837, 12.8981)
  line L1578 (-4.1837, 12.8981) -> (-4.1616, 12.9808)
  line L1579 (3.7733, -2.0203) -> (3.6906, -1.9981)
  line L1580 (3.6906, -1.9981) -> (3.6079, -2.0203)
  line L1581 (3.6079, -2.0203) -> (3.5474, -2.0808)
  line L1582 (3.5474, -2.0808) -> (3.5253, -2.1635)
  line L1583 (3.5253, -2.1635) -> (3.5474, -2.2461)
  line L1584 (3.5474, -2.2461) -> (3.6079, -2.3067)
  line L1585 (3.6079, -2.3067) -> (3.6906, -2.3288)
  line L1586 (3.6906, -2.3288) -> (3.7733, -2.3067)
  line L1587 (3.7733, -2.3067) -> (3.8338, -2.2461)
  line L1588 (3.8338, -2.2461) -> (3.856, -2.1635)
  line L1589 (-1.2345, 8.5266) -> (-1.2567, 8.6093)
  line L1590 (-1.2567, 8.6093) -> (-1.3172, 8.6698)
  line L1591 (-1.3172, 8.6698) -> (-1.3999, 8.6919)
  line L1592 (-1.4826, 8.6698) -> (-1.5431, 8.6093)
  line L1593 (-1.5431, 8.6093) -> (-1.5652, 8.5266)
  line L1594 (-1.5652, 8.5266) -> (-1.5431, 8.4439)
  line L1595 (-1.5431, 8.4439) -> (-1.4826, 8.3834)
  line L1596 (-1.4826, 8.3834) -> (-1.3999, 8.3613)
  line L1597 (-1.3999, 8.3613) -> (-1.3172, 8.3834)
  line L1598 (-1.3172, 8.3834) -> (-1.2567, 8.4439)
  line L1599 (-1.2567, 8.4439) -> (-1.2345, 8.5266)
  line L1600 (-15.1823, 7.254) -> (-15.1602, 7.1713)
  line L1601 (-15.1602, 7.1713) -> (-15.0997, 7.1108)
  line L1602 (-15.0997, 7.1108) -> (-15.017, 7.0886)
  line L1603 (-15.017, 7.0886) -> (-14.9343, 7.1108)
  line L1604 (-14.9343, 7.1108) -> (-14.8738, 7.1713)
  line L1605 (-15.2335, -0.6363) -> (-15.2556, -0.5536)
  line L1606 (-15.2556, -0.5536) -> (-15.3161, -0.4931)
  line L1607 (-15.3161, -0.4931) -> (-15.3988, -0.471)
  line L1608 (-15.3988, -0.471) -> (-15.4815, -0.4931)
  line L1609 (-15.4815, -0.4931) -> (-15.542, -0.5536)
  line L1610 (-15.542, -0.5536) -> (-15.5641, -0.6363)
  line L1611 (-15.5641, -0.6363) -> (-15.542, -0.719)
  line L1612 (-15.542, -0.719) -> (-15.4815, -0.7795)
  line L1613 (-15.4815, -0.7795) -> (-15.3988, -0.8017)
  line L1614 (-15.3988, -0.8017) -> (-15.3161, -0.7795)
  line L1615 (-15.3161, -0.7795) -> (-15.2556, -0.719)
  line L1616 (-15.2556, -0.719) -> (-15.2335, -0.6363)
  line L1617 (13.5279, 2.1635) -> (13.5058, 2.2461)
  line L1618 (13.5058, 2.2461) -> (13.4453, 2.3067)
  line L1619 (13.4453, 2.3067) -> (13.3626, 2.3288)
  line L1620 (13.3626, 2.3288) -> (13.2799, 2.3067)
  line L1621 (13.2799, 2.3067) -> (13.2194, 2.2461)
  line L1622 (13.2194, 2.2461) -> (13.1972, 2.1635)
  line L1623 (13.1972, 2.1635) -> (13.2194, 2.0808)
  line L1624 (14.8006, 2.418) -> (14.7784, 2.5007)
  line L1625 (14.7784, 2.5007) -> (14.7179, 2.5612)
  line L1626 (14.7179, 2.5612) -> (14.6352, 2.5833)
  line L1627 (14.6352, 2.5833) -> (14.5525, 2.5612)
  line L1628 (14.5525, 2.5612) -> (14.492, 2.5007)
  line L1629 (14.492, 2.5007) -> (14.4699, 2.418)
  line L1630 (14.4699, 2.418) -> (14.492, 2.3353)
  line L1631 (14.5525, 2.2748) -> (14.6352, 2.2527)
  line L1632 (14.6352, 2.2527) -> (14.7179, 2.2748)
  line L1633 (14.7179, 2.2748) -> (14.7784, 2.3353)
  line L1634 (-2.5072, 3.6906) -> (-2.5293, 3.7733)
  line L1635 (-2.5293, 3.7733) -> (-2.5898, 3.8338)
  line L1636 (-2.5898, 3.8338) -> (-2.6725, 3.856)
  line L1637 (-2.6725, 3.856) -> (-2.7552, 3.8338)
  line L1638 (-2.7552, 3.8338) -> (-2.8157, 3.7733)
  line L1639 (-2.8157, 3.7733) -> (-2.8379, 3.6906)
  line L1640 (-2.8379, 3.6906) -> (-2.8157, 3.6079)
  line L1641 (-2.8157, 3.6079) -> (-2.7552, 3.5474)
  line L1642 (-2.7552, 3.5474) -> (-2.6725, 3.5253)
  line L1643 (-0.7255, 3.6906) -> (-0.7476, 3.7733)
  line L1644 (-0.7476, 3.7733) -> (-0.8082, 3.8338)
  line L1645 (-0.8082, 3.8338) -> (-0.8908, 3.856)
  line L1646 (-0.8908, 3.856) -> (-0.9735, 3.8338)
  line L1647 (-0.9735, 3.8338) -> (-1.034, 3.7733)
  line L1648 (-1.034, 3.7733) -> (-1.0562, 3.6906)
  line L1649 (-1.0562, 3.6906) -> (-1.034, 3.6079)
  line L1650 (-1.034, 3.6079) -> (-0.9735, 3.5474)
  line L1651 (-0.9735, 3.5474) -> (-0.8908, 3.5253)
  line L1652 (-0.8908, 3.5253) -> (-0.8082, 3.5474)
  line L1653 (-0.7476, 3.6079) -> (-0.7255, 3.6906)
  line L1654 (11.2372, -2.1635) -> (11.215, -2.0808)
  line L1655 (11.215, -2.0808) -> (11.1545, -2.0203)
  line L1656 (11.1545, -2.0203) -> (11.0719, -1.9981)
  line L1657 (11.0719, -1.9981) -> (10.9892, -2.0203)
  line L1658 (10.9892, -2.0203) -> (10.9287, -2.0808)
  line L1659 (10.9287, -2.0808) -> (10.9065, -2.1635)
  line L1660 (10.9065, -2.1635) -> (10.9287, -2.2461)
  line L1661 (10.9287, -2.2461) -> (10.9892, -2.3067)
  line L1662 (10.9892, -2.3067) -> (11.0719, -2.3288)
  line L1663 (11.0719, -2.3288) -> (11.1545, -2.3067)
  line L1664 (11.1545, -2.3067) -> (11.215, -2.2461)
  line L1665 (11.215, -2.2461) -> (11.2372, -2.1635)
  line L1666 (8.0176, 7.763) -> (7.9835, 7.8903)
  line L1667 (7.9835, 7.8903) -> (7.8903, 7.9835)
  line L1668 (7.8903, 7.9835) -> (7.763, 8.0176)
  line L1669 (7.763, 8.0176) -> (7.6358, 7.9835)
  line L1670 (7.6358, 7.9835) -> (7.5426, 7.8903)
  line L1671 (7.5426, 7.8903) -> (7.5085, 7.763)
  line L1672 (7.5085, 7.763) -> (7.5426, 7.6358)
  line L1673 (7.5426, 7.6358) -> (7.6358, 7.5426)
  line L1674 (7.6358, 7.5426) -> (7.763, 7.5085)
  line L1675 (7.763, 7.5085) -> (7.8903, 7.5426)
  line L1676 (7.8903, 7.5426) -> (7.9835, 7.6358)
  line L1677 (7.9835, 7.6358) -> (8.0176, 7.763)
  line L1678 (-7.5085, -7.763) -> (-7.5426, -7.6358)
  line L1679 (-7.5426, -7.6358) -> (-7.6358, -7.5426)
  line L1680 (-7.6358, -7.5426) -> (-7.763, -7.5085)
  line L1681 (-7.763, -7.5085) -> (-7.8903, -7.5426)
  line L1682 (-7.9835, -7.6358) -> (-8.0176, -7.763)
  line L1683 (-8.0176, -7.763) -> (-7.9835, -7.8903)
  line L1684 (-7.9835, -7.8903) -> (-7.8903, -7.9835)
  line L1685 (-7.8903, -7.9835) -> (-7.763, -8.0176)
  line L1686 (-7.763, -8.0176) -> (-7.6358, -7.9835)
  line L1687 (-7.6358, -7.9835) -> (-7.5426, -7.8903)
  line L1688 (-7.5426, -7.8903) -> (-7.5085, -7.763)
  line L1689 (-13.3626, 18.4531) -> (-13.6955, 18.4422)
  line L1690 (-13.6955, 18.4422) -> (-14.027, 18.4096)
  line L1691 (-14.027, 18.4096) -> (-14.3557, 18.3553)
  line L1692 (-14.3557, 18.3553) -> (-14.6801, 18.2796)
  line L1693 (-14.9989, 18.1829) -> (-15.3106, 18.0656)
  line L1694 (-15.3106, 18.0656) -> (-15.6141, 17.9281)
  line L1695 (-15.6141, 17.9281) -> (-15.9078, 17.7711)
  line L1696 (-15.9078, 17.7711) -> (-16.1907, 17.5952)
  line L1697 (-16.1907, 17.5952) -> (-16.4615, 17.4012)
  line L1698 (-16.4615, 17.4012) -> (-16.719, 17.1898)
  line L1699 (-16.719, 17.1898) -> (-16.9621, 16.9621)
  line L1700 (-16.9621, 16.9621) -> (-17.1898, 16.719)
  line L1701 (-17.1898, 16.719) -> (-17.4012, 16.4615)
  line L1702 (-17.4012, 16.4615) -> (-17.5952, 16.1907)
  line L1703 (-17.7711, 15.9078) -> (-17.9281, 15.6141)
  line L1704 (-17.9281, 15.6141) -> (-18.0656, 15.3106)
  line L1705 (-18.1829, 14.9989) -> (-18.2796, 14.6801)
  line L1706 (-18.2796, 14.6801) -> (-18.3553, 14.3557)
  line L1707 (-18.3553, 14.3557) -> (-18.4095, 14.027)
  line L1708 (-18.4095, 14.027) -> (-18.4422, 13.6955)
  line L1709 (-18.4422, 13.6955) -> (-18.4531, 13.3626)
  line L1710 (-18.4531, -14.2304) -> (-18.4528, -14.5799)
  dimension "d2" = 36.9062
  constraints: 3422 end point
  measures "d2" distance between parallel lines of L253 L111
extrude "Extrusion1" add sketch "PCB" along normal blind 0.6604
move or copy body "Move Body1" bodies to move or copy 1 copy no rotation origin (0, 0, 0) rotation axis (-0.5773503, -0.5773503, 0.5773503) rotation angle -120
sketch "Sketch3" plane through (-6.6988, 0, 18.4531) normal (0, 1, 0) x (1, 0, 0)
  line L0 (25.1232, 36.8974) -> (25.1232, 0.0469) construction
  line L1 (25.1232, 0.0469) -> (-11.7272, 0.0469) construction
  line L2 (-11.7272, 0.0469) -> (-11.7272, 36.8974) construction
  line L3 (-11.7272, 36.8974) -> (25.1232, 36.8974) construction
  point P0 (6.6988, 18.4531)
  constraints: 2 other
sketch "Sketch4" plane through (-6.6988, -0.6604, 18.4531) normal (0, -1, 0) x (1, 0, 0)
  line L0 (25.1481, -0.0234) -> (25.1481, -36.8738) construction
  line L1 (25.1481, -36.8738) -> (-11.7024, -36.8738) construction
  line L2 (-11.7024, -36.8738) -> (-11.7024, -0.0234) construction
  line L3 (-11.7024, -0.0234) -> (25.1481, -0.0234) construction
  point P0 (6.6988, -18.4531)
  constraints: 2 other
decal "Decal1"
decal "Decal2"
body "Solid1"
